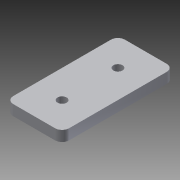
# Autodesk Inventor part: Spacer
Saved by Autodesk Inventor 2014 (Build 180170000, 170)
## iProperties
Created: 2014-01-05
Part Number: Spacer
Material: Aluminum 6061
Document SubType Name: Modeling
Designer: Andrew Toennies
Mass: 16.1899 g
Surface Area: 33.3332 cm^2
Volume: 5.97413 cm^3
Density: 2.71 g/cm^3
Appearance: Aluminum - Flat
Author: Andrew Toennies
Autodesk Inventor part; units mm, degrees
ref_plane "YZ Plane" through (0, 0, 0) normal (1, 0, 0) x (0, 1, 0)
ref_plane "XZ Plane" through (0, 0, 0) normal (0, 1, 0) x (-1, 0, 0)
ref_plane "XY Plane" through (0, 0, 0) normal (0, 0, 1) x (1, 0, 0)
sketch "Sketch1" plane through (0, 0, 0) normal (0, 1, 0) x (-1, 0, 0)
  line L0 (0, 0) -> (25.4, 0)
  line L1 (25.4, 0) -> (25.4, 50.8)
  line L2 (25.4, 50.8) -> (0, 50.8)
  line L3 (0, 50.8) -> (0, 0)
  dimension "d0" = 25.4
  dimension "d1" = 50.8
  constraints: 8 end point, 2 parallel, 1 horizontal, 1 perpendicular
  measures "d0" distance of L1.end L2.end
  measures "d1" distance of L0.end L1.end
extrude "Extrusion1" add sketch "Sketch1" along normal blind 4.7625
sketch "Sketch2" plane through (0, 4.7625, 0) normal (0, 1, 0) x (1, 0, 0)
  line L0 (0, 0) -> (-25.4, 0) projected
  line L1 (0, -50.8) -> (0, 0) projected
  circle A0 centre (-12.7, -12.7) radius 2.0828
  dimension "d5" = 4.1656
  dimension "d6" = 12.7
  dimension "d7" = 12.7
  constraints: 1 centre point
  measures "d5" diameter of A0
  measures "d6" distance from line of L1 A0.centre
  measures "d7" distance from line of L0 A0.centre
extrude "Extrusion2" cut sketch "Sketch2" against normal blind 4.7625
pattern_linear "Rectangular Pattern1" count 2 spacing 25.4 along (0, 0, 1) of "Extrusion2"
fillet "Fillet1" radius 3.175 4 edges at (0, 2.3813, 50.8) (-25.4, 2.3813, 50.8) (-25.4, 2.3813, 0) (0, 2.3813, 0)
body "Solid1"
